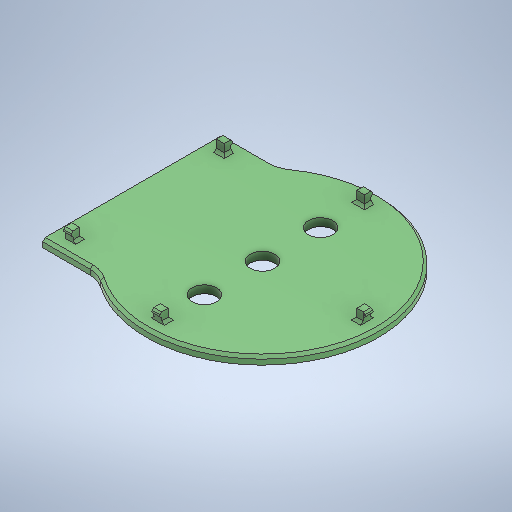
# Autodesk Inventor part: SCARA arm base - lid
Saved by Autodesk Inventor 2025.2 (Build 292293000, 293)
## iProperties
Created: 2025-01-29
Part Number: SCARA arm base - lid
Material: Generic
Document SubType Name: Modeling
Designer: caomi
Density: 1 g/cm^3
Appearance: Default
Author: caomi
Autodesk Inventor part; units mm, degrees
ref_plane "YZ Plane" through (0, 0, 0) normal (1, 0, 0) x (0, 1, 0)
ref_plane "XZ Plane" through (0, 0, 0) normal (0, 1, 0) x (-1, 0, 0)
ref_plane "XY Plane" through (0, 0, 0) normal (0, 0, 1) x (1, 0, 0)
sketch "Sketch1" plane through (0, 0, 0) normal (0, 1, 0) x (-1, 0, 0)
  circle A0 centre (0, 0) radius 45
  line L0 (28.2843, 35) -> (50, 35)
  line L1 (50, 35) -> (50, -35)
  line L2 (50, -35) -> (28.2843, -35)
  dimension "d0" = 90
  dimension "d1" = 70
  dimension "d2" = 50
  constraints: 6 end point, 2 perpendicular, 2 point on circle, 1 centre point, 1 coincident, 1 horizontal, 1 vertical alignment
  measures "d0" diameter of A0
  measures "d1" distance of L0.end L1.end
  measures "d2" distance from line of point (0, 0) L1
extrude "Extrusion1" add sketch "Sketch1" along normal blind 3
fillet "Fillet1" radius 10 2 edges at (-28.2843, 1.5, 35) (-28.2843, 1.5, -35)
sketch "Sketch3" plane through (0, 3, 0) normal (0, 1, 0) x (1, 0, 0)
  circle A0 centre (0, 0) radius 4.75
  circle A1 centre (0, -22.5) radius 4.75
  circle A2 centre (0, 22.5) radius 4.75
  line L0 (-69, 0) -> (64, 0) projected
  dimension "d16" = 45
  dimension "d17" = 9.5
  constraints: 3 centre point, 2 equal radius, 1 coincident, 1 symmetric about line, 1 vertical alignment
  measures "d16" distance of A2.centre A1.centre
  measures "d17" diameter of A0
extrude "Extrusion2" cut sketch "Sketch3" against normal blind 9.5
sketch "Sketch5" plane through (0, 3, 0) normal (0, 1, 0) x (1, 0, 0)
  arc A0 (-25.8732, -36.8182) -> (-25.8732, 36.8182) centre (0, 0) ccw projected
  arc A1 (-25.8732, -36.8182) -> (-31.6228, -35) centre (-31.6228, -45) ccw projected
  line L0 (-50, -35) -> (-31.6228, -35) projected
  line L1 (-50, 35) -> (-50, -35) projected
  line L2 (-31.6228, 35) -> (-50, 35) projected
  arc A2 (-31.6228, 35) -> (-25.8732, 36.8182) centre (-31.6228, 45) ccw projected
  arc A3 (-23.2859, -33.1364) -> (-23.2859, 33.1364) centre (0, 0) ccw
  arc A4 (-23.2859, -33.1364) -> (-31.6228, -30.5) centre (-31.6228, -45) ccw
  line L3 (-31.6228, -30.5) -> (-45.5, -30.5)
  line L4 (-45.5, -30.5) -> (-45.5, 30.5)
  line L5 (-45.5, 30.5) -> (-31.6228, 30.5)
  arc A5 (-31.6228, 30.5) -> (-23.2859, 33.1364) centre (-31.6228, 45) ccw
  arc A6 (-21.8485, -31.0909) -> (-21.8485, 31.0909) centre (0, 0) ccw
  arc A7 (-21.8485, -31.0909) -> (-31.6228, -28) centre (-31.6228, -45) ccw
  line L6 (-31.6228, -28) -> (-43, -28)
  line L7 (-43, -28) -> (-43, 28)
  line L8 (-43, 28) -> (-31.6228, 28)
  arc A8 (-31.6228, 28) -> (-21.8485, 31.0909) centre (-31.6228, 45) ccw
  line L9 (37.9704, -1.5) -> (40.4722, -1.5)
  line L10 (37.9704, 1.5) -> (40.4722, 1.5)
  line L11 (0, 0) -> (25.5499, 0) construction
  line L12 (-42.8, -30.5) -> (-42.8, -28)
  line L13 (-45.8, -30.5) -> (-45.8, -28)
  line L14 (-45.8, -28) -> (-42.8, -28)
  line L15 (-45.8, -30.5) -> (-42.8, -30.5)
  point P0 (-45.5, -28)
  dimension "d20" = 4.5
  dimension "d21" = 2.5
  dimension "d22" = 3
  dimension "d33" = 3
  dimension "d51" = 0.3
  constraints: 26 end point, 16 point on circle, 6 centre point, 4 point on line, 3 horizontal, 2 collinear, 1 perpendicular, 1 vertical, 11 other
  measures "d20" radial gap between concentric circles of A0 A3
  measures "d21" radial gap between concentric circles of A3 A6
  measures "d22" distance between parallel lines of L9 L10
  measures "d33" distance between parallel lines of L13 L12
  measures "d51" distance between parallel lines of L4 L13
extrude "Extrusion3" add sketch "Sketch5" along normal blind 4 contours L9 A6 L10 A3
sketch "Sketch6" plane through (40.4722, 3, -1.5) normal (0, 0, -1) x (-1, 0, 0)
  line L0 (0, 4) -> (-1, 3)
  line L1 (-1, 3) -> (0, 2)
  line L2 (-1, 3) -> (-1.2746, 3) construction
  line L3 (0, 0) -> (0, 4) projected
  line L4 (0, 4) -> (0, 2)
  point P0 (40.4722, -3)
  dimension "d26" = 45
  dimension "d27" = 1
  constraints: 8 end point, 1 horizontal, 1 midpoint, 1 other
  measures "d26" angle of L1 L2
  measures "d27" distance from line of L3 L0.end
sketch3d "3D Sketch1"
  arc A0 (40.4722, 7, -1.5) -> (40.4722, 7, 1.5) centre (0, 7, 0) ccw
sweep "Sweep1" add profiles "Sketch6" path "3D Sketch1"
pattern_circular "Circular Pattern1" count 2 over 90 about axis through (0, 0, 0) along (0, -1, 0) of "Sweep1", "Extrusion3"
extrude "Extrusion5" add sketch "Sketch5" along normal up to surface (4 mm away) contours L9 A6 L10 A3 | L3 L4 L14 L6 L12 | L15 L13 L14 L4
sketch "Sketch7" plane through (-42.8, 3, 30.5) normal (1, 0, 0) x (0, 0, -1)
  line L0 (-1, 3) -> (0.0311, 1.9689)
  line L1 (-1.364, 3) -> (-0.0782, 3) construction
  line L2 (0, 0) -> (0, 4) projected
  line L3 (-1, 3) -> (0, 4)
  point P0 (30.5, -3)
  point P1 (0, 2)
  dimension "d36" = 45
  dimension "d42" = 1
  constraints: 6 end point, 1 horizontal, 1 point on line, 1 other
  measures "d36" angle of L1 L0
  measures "d42" distance from line of L0.start L2
extrude "Extrusion4" add sketch "Sketch7" against normal up to surface (3 mm away)
chamfer "Chamfer1" distance 1 angle 45 8 edges at (-42.8, 3, 29.25) (1.5, 3, 39.2213) (0, 3, 38) (-1.5, 3, 39.2213) (38, 3, 0) (39.2213, 3, 1.5) (39.2213, 3, -1.5) (-44.3, 3, 28)
fillet "Fillet2" radius 0.5 3 edges at (41.4993, 6, 0.037) (-0.037, 6, 41.4993) (-44.3, 6, 31.5)
mirror "Mirror1" about plane through (0, 0, 0) normal (0, 0, 1) of "Sweep1", "Extrusion3", "Circular Pattern1", "Extrusion4", "Extrusion5", "Chamfer1", "Fillet2"
chamfer "Chamfer2" distance 1 angle 45 5 edges at (45, 3, 0) (-28.6077, 3, -35.4654) (-40.8114, 3, -35) (-28.6077, 3, 35.4654) (-40.8114, 3, 35)
equation "\"d18\" = d17"
equation "\"d33\" = d22"
equation "\"d42\" = d27"
body "Solid1"
